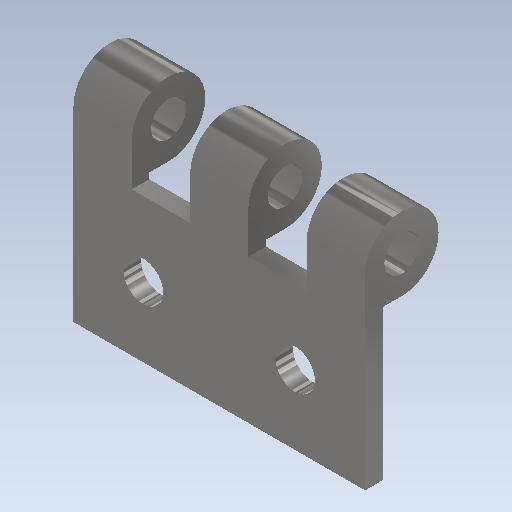
# Autodesk Inventor part: 2HHKS25
Saved by Autodesk Inventor 2021 (Build 250183000, 183)
## iProperties
Part Number: 2HHKS25
Material: ステンレス鋼
Catalog Web Link: www.cadenas.de
Description: HHKS-2-Hinges
Vendor: MISUMI
Document SubType Name: Modeling
Designer: partserver
Manufacturer: MISUMI
Mass: 6.72509 g
Surface Area: 13.1571 cm^2
Volume: 0.840636 cm^3
Density: 8 g/cm^3
Appearance: 半つや出し
Category: PARTsolutions
Company: MISUMI
PSOL_IDENT_0: {$CADENAS_DATA\23d-libs\misumi\metric\43_levers_knobs\parts_hhks\hhks_2.prj},147 {VTYP=3D},{NB=2HHKS
PSOL_IDENT_1: 25},{LINA=2HHKS25},{NN=HHKS-2},{DATE=30.03.2018 07:16:18},{GEOMDATE=17.02.2014},{VERSION=},{LINEID=1
PSOL_IDENT_2: 0},{WBVAR=L},{WBNUMERIC=L}  {NB=2HHKS25},{LINA=2HHKS25},{KT=DUMMY},{PN=HHKS25},{MAT=304 Stainless St
PSOL_IDENT_3: eel},{L=25},{LL=6.0},{L1=13},{L2=0},{L3=0},{NOD=3},{AL=29.4},{WEIGHT=13}
NB: 2HHKS25
NN: HHKS-2
NT: Hinges
NBSYN: 2$PN.
LINA: 2HHKS25
CATALOG: Misumi
MAT: 304 Stainless Steel
L: 25
SUPPLIER: MISUMI
ARTICLENO: 2HHKS25
BOMINFO: 2HHKS25
CREATOR: CADENAS GmbH
Title: 2HHKS25
Author: Cadenas PARTsolutions
Comments: Hinges
Autodesk Inventor part; units mm, degrees
sketch "Sketch_1" plane through (0, 0, 0) normal (0, 1, 0) x (-1, 0, 0)
  line L0 (0, 16) -> (-25, 16)
  line L1 (-25, 16) -> (-25, 3.15)
  line L2 (-25, 3.15) -> (-20, 3.15)
  line L3 (-20, 3.15) -> (-20, 3.65)
  line L4 (-20, 3.65) -> (-15, 3.65)
  line L5 (-15, 3.65) -> (-15, 3.15)
  line L6 (-15, 3.15) -> (-10, 3.15)
  line L7 (-10, 3.15) -> (-10, 3.65)
  line L8 (-10, 3.65) -> (-5, 3.65)
  line L9 (-5, 3.65) -> (-5, 3.15)
  line L10 (-5, 3.15) -> (0, 3.15)
  line L11 (0, 3.15) -> (0, 16)
  constraints: 24 end point
extrude "Extrusion1" add sketch "Sketch_1" along normal blind 1.5
sketch "Sketch_2" plane through (0, 0, 0) normal (1, 0, 0) x (0, 1, 0)
  line L0 (1.5, 10.6667) -> (0, 10.6667)
  line L1 (0, 10.6667) -> (0, 0)
  arc A0 (0, 0) -> (3.15, 3.15) centre (3.15, 0) ccw
  line L2 (3.15, 3.15) -> (1.5, 3.15)
  line L3 (1.5, 3.15) -> (1.5, 10.6667)
  circle A1 centre (3.15, 0) radius 1.5
  constraints: 8 end point, 2 centre point, 2 point on circle
extrude "Extrusion2" add sketch "Sketch_2" along normal blind 5
sketch "Sketch_3" plane through (10, 0, 0) normal (1, 0, 0) x (0, 0, -1)
  line L0 (-10.6667, 1.5) -> (-10.6667, 0)
  line L1 (-10.6667, 0) -> (0, 0)
  arc A0 (0, 0) -> (-3.15, 3.15) centre (0, 3.15) ccw
  line L2 (-3.15, 3.15) -> (-3.15, 1.5)
  line L3 (-3.15, 1.5) -> (-10.6667, 1.5)
  circle A1 centre (0, 3.15) radius 1.5
  constraints: 8 end point, 2 centre point, 2 point on circle
extrude "Extrusion3" add sketch "Sketch_3" along normal blind 5
sketch "Sketch_4" plane through (20, 0, 0) normal (1, 0, 0) x (0, 0, -1)
  line L0 (-10.6667, 1.5) -> (-10.6667, 0)
  line L1 (-10.6667, 0) -> (0, 0)
  arc A0 (0, 0) -> (-3.15, 3.15) centre (0, 3.15) ccw
  line L2 (-3.15, 3.15) -> (-3.15, 1.5)
  line L3 (-3.15, 1.5) -> (-10.6667, 1.5)
  circle A1 centre (0, 3.15) radius 1.5
  constraints: 8 end point, 2 centre point, 2 point on circle
extrude "Extrusion4" add sketch "Sketch_4" along normal blind 5
sketch "Sketch5" plane through (0, 0, 0) normal (0, -1, 0) x (1, 0, 0)
  point P0 (6, 10)
hole "Hole1" at (6, 0, 10) direction (0, 1, 0) diameter 3.4 depth 2
sketch "Sketch6" plane through (0, 0, 0) normal (0, -1, 0) x (1, 0, 0)
  point P0 (19, 10)
hole "Hole2" at (19, 0, 10) direction (0, 1, 0) diameter 3.4 depth 2
ref_plane "2_XY" through (0, 3.15, 0) normal (1, 0, 0) x (0, 0, -1)
ref_plane "2_YZ" through (0, 3.15, 0) normal (0, 0, -1) x (0, 1, 0)
ref_plane "2_ZX" through (0, 3.15, 0) normal (0, 1, 0) x (1, 0, 0)
body "Solid1"
